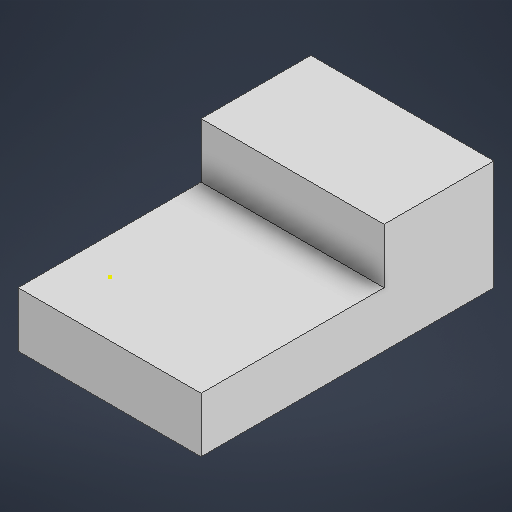
# Autodesk Inventor part: Part3
Saved by Autodesk Inventor 2026 (Build 300175050, 175E)
## iProperties
Created: 2026-03-12
Part Number: Part3
Material: Generic
Document SubType Name: Modeling
Designer: Administrator
Density: 1 g/cm^3
Appearance: Default
Author: Administrator
Autodesk Inventor part; units mm, degrees
ref_plane "YZ Plane" through (0, 0, 0) normal (1, 0, 0) x (0, 1, 0)
ref_plane "XZ Plane" through (0, 0, 0) normal (0, 1, 0) x (-1, 0, 0)
ref_plane "XY Plane" through (0, 0, 0) normal (0, 0, 1) x (1, 0, 0)
sketch "Sketch1" plane through (0, 0, 0) normal (1, 0, 0) x (0, 1, 0)
  line L0 (0, 0) -> (15, 0)
  line L1 (15, 0) -> (15, -40)
  line L2 (15, -40) -> (0, -40)
  line L3 (0, -40) -> (0, 0)
  dimension "d0" = 40
  dimension "d1" = 15
  constraints: 8 end point, 2 parallel, 1 horizontal, 1 perpendicular
  measures "d0" distance of L0.end L1.end
  measures "d1" distance of L1.end L2.end
extrude "Extrusion1" add sketch "Sketch1" along normal mid plane 25
sketch "Sketch2" plane through (12.5, 0, 0) normal (1, 0, 0) x (0, 0, -1)
  line L0 (-5, 16.2216) -> (25, 16.2216)
  line L1 (25, 16.2216) -> (25, 7.5)
  line L2 (25, 7.5) -> (-5, 7.5)
  line L3 (-5, 7.5) -> (-5, 16.2216)
  line L4 (40, 0) -> (40, 15) projected
  line L5 (0, 0) -> (40, 0) projected
  dimension "d4" = 15
  dimension "d5" = 30
  dimension "d6" = 7.5
  constraints: 8 end point, 2 parallel, 1 horizontal, 1 perpendicular
  measures "d4" distance between parallel lines of L4 L1
  measures "d5" distance of L1.end L2.end
  measures "d6" distance between parallel lines of L5 L2
extrude "Extrusion2" cut sketch "Sketch2" against normal through all
sketch "Sketch3" plane through (-12.5, 15, -40) normal (0, 1, 0) x (1, 0, 0)
  point P0 (12.5, -40)
body "Solid1"
